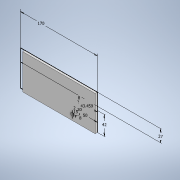
# Autodesk Inventor part: Inkpath_Plate
Saved by Autodesk Inventor 2022 (Build 260153000, 153)
## iProperties
Created: 2024-04-03
Part Number: Inkpath_Plate
Material: Generic
Document SubType Name: Modeling
Designer: Gotham City
Density: 1 g/cm^3
Appearance: Default
Author: Gotham City
Autodesk Inventor part; units mm, degrees
ref_plane "YZ Plane" through (0, 0, 0) normal (1, 0, 0) x (0, 1, 0)
ref_plane "XZ Plane" through (0, 0, 0) normal (0, 1, 0) x (-1, 0, 0)
ref_plane "XY Plane" through (0, 0, 0) normal (0, 0, 1) x (1, 0, 0)
sketch "Sketch1" plane through (0, 0, 0) normal (0, 0, 1) x (1, 0, 0)
  line L0 (0, 0) -> (-170, 0)
  line L1 (-170, 0) -> (-170, -50)
  line L2 (-170, -50) -> (0, -50)
  line L3 (0, -50) -> (0, 0)
  line L4 (0, 0) -> (-43.459, 0)
  line L5 (-43.459, 0) -> (-43.459, -8)
  line L6 (-43.459, -8) -> (0, -8)
  line L7 (0, -8) -> (0, 0)
  line L8 (0, 0) -> (-170, 0)
  line L9 (-170, 0) -> (-170, 27)
  line L10 (-170, 27) -> (0, 27)
  line L11 (0, 27) -> (0, 0)
  circle A0 centre (-50, -38) radius 4
  line L12 (-51, -30.5) -> (-49, -30.5)
  line L13 (-49, -30.5) -> (-49, -45.5)
  line L14 (-49, -45.5) -> (-51, -45.5)
  line L15 (-51, -45.5) -> (-51, -30.5)
  line L16 (-50, -38) -> (-50, -42) construction
  line L17 (-51, -38) -> (-50, -38) construction
  point P0 (-51, -34.127)
  point P1 (-51, -41.873)
  point P2 (-49, -34.127)
  point P3 (-49, -41.873)
  dimension "d10" = 8
  dimension "d0" = 43.459
  dimension "d1" = 8
  dimension "d2" = 27
  dimension "d3" = 42
  dimension "d4" = 170
  dimension "d8" = 30
  dimension "d9" = 50
  dimension "d11" = 15
  dimension "d12" = 2
  constraints: 36 end point, 8 parallel, 5 horizontal, 4 perpendicular, 1 midpoint, 1 vertical, 4 other
  measures "d0" distance of L5.end L6.end
  measures "d1" distance of L4.end L5.end
  measures "d2" distance of L0.end L9.end
  measures "d3" distance between parallel lines of L2 L6
  measures "d4" distance between parallel lines of L3 L1
  measures "d8" distance from line of L16.start L6
  measures "d9" distance from line of L3 L16.start
  measures "d11" distance of L12.end L13.end
  measures "d12" distance of L12.start L12.end
sketch "Sketch2" plane through (0, 0, 0) normal (0, 0, 1) x (1, 0, 0)
  line L0 (0, 27) -> (-160, 27)
  line L1 (-160, 27) -> (-160, -50)
  line L2 (-160, -50) -> (0, -50)
  line L3 (0, -50) -> (0, 27)
  point P0 (0, 0)
  dimension "d5" = 160
  constraints: 8 end point, 2 parallel, 1 horizontal, 1 perpendicular, 1 point on line
  measures "d5" distance of L1.end L2.end
extrude "Extrusion1" add sketch "Sketch2" along normal blind 5
extrude "Extrusion2" cut sketch "Sketch1" along normal through all contours A0 L13 | L13 A0 L15 | A0 L15 L12 L13 | L13 L14 L15 A0 | L15 A0
body "Solid1"
